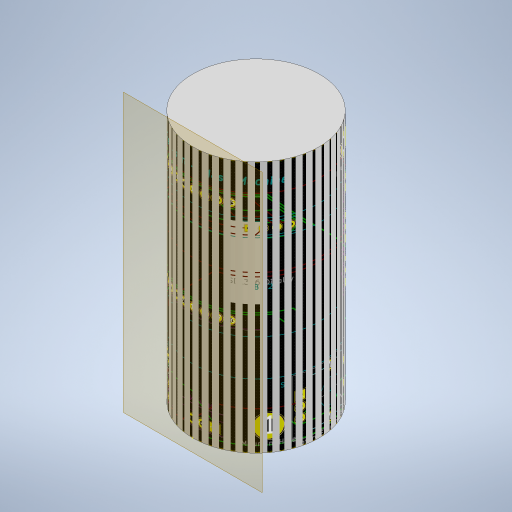
# Autodesk Inventor part: understanding images and decals
Saved by Autodesk Inventor 2024 (Build 280153000, 153)
## iProperties
Created: 2024-11-04
Part Number: understanding images and decals
Material: Generic
Document SubType Name: Modeling
Designer: Emil
Density: 1 g/cm^3
Appearance: Default
Author: Emil
Autodesk Inventor part; units mm, degrees
ref_plane "YZ Plane" through (0, 0, 0) normal (1, 0, 0) x (0, 1, 0)
ref_plane "XZ Plane" through (0, 0, 0) normal (0, 1, 0) x (-1, 0, 0)
sketch "Sketch3" plane through (0, 0, 0) normal (0, 1, 0) x (-1, 0, 0)
  circle A0 centre (0, 0) radius 5
  dimension "d7" = 10
  constraints: 1 centre point, 1 coincident
  measures "d7" diameter of A0
extrude "Extrusion1" add sketch "Sketch3" along normal blind 20
ref_plane "Work Plane1" through (0, 0, 5) normal (0, 0, 1) x (1, 0, 0)
sketch "Sketch4" plane through (0, 0, 5) normal (0, 0, 1) x (1, 0, 0)
  line L0 (-12.9248, 20) -> (12.9248, 20) construction
  line L1 (12.9248, 20) -> (12.9248, 0) construction
  line L2 (12.9248, 0) -> (-12.9248, 0) construction
  line L3 (-12.9248, 0) -> (-12.9248, 20) construction
  line L4 (5, 20) -> (-5, 20) projected
  line L5 (5, 0) -> (-5, 0) projected
  line L6 (-5, 20) -> (5, 20)
  line L7 (5, 20) -> (5, 0)
  line L8 (5, 0) -> (-5, 0)
  line L9 (-5, 0) -> (-5, 20)
  line L10 (-12.9248, 20) -> (12.9248, 20)
  line L11 (12.9248, 20) -> (12.9248, 0)
  line L12 (12.9248, 0) -> (-12.9248, 0)
  line L13 (-12.9248, 0) -> (-12.9248, 20)
  line L14 (0, 20) -> (0, 0)
  constraints: 18 end point, 4 parallel, 3 perpendicular, 2 collinear, 2 horizontal, 1 midpoint, 3 other
decal "Decal1"
sketch "Sketch5" plane through (0, 0, 5) normal (0, 0, 1) x (1, 0, 0)
  point P0 (0, 0)
body "Solid1"
